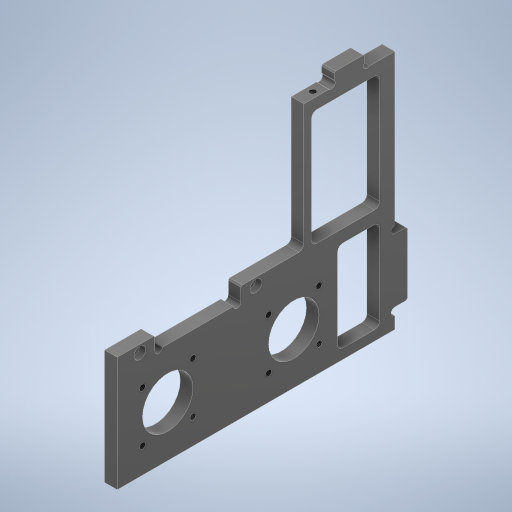
# Autodesk Inventor part: TorsoElectronicBoxSideFrame_
Saved by Autodesk Inventor 2024.2 (Build 282272000, 272)
## iProperties
Created: 2024-01-27
Part Number: TorsoElectronicBoxSideFrame_
Material: Acetal Resin, Black
Document SubType Name: Modeling
Designer: Masato Kubotera
Density: 1.425 g/cm^3
Appearance: Smooth - Black
Vendor: meviy
Mass: 39.5202 g
Surface Area: 148.13 cm^2
Volume: 27.7334 cm^3
Author: Masato Kubotera
Autodesk Inventor part; units mm, degrees
ref_plane "YZ Plane" through (0, 0, 0) normal (1, 0, 0) x (0, 1, 0)
ref_plane "XZ Plane" through (0, 0, 0) normal (0, 1, 0) x (-1, 0, 0)
ref_plane "XY Plane" through (0, 0, 0) normal (0, 0, 1) x (1, 0, 0)
derived "TorsoSideFrame_.ipt"
sketch "Sketch1" plane through (0, 0, 0) normal (0, 1, 0) x (-1, 0, 0)
  circle A0 centre (0, 0) radius 18.75
  line L0 (0, 0) -> (0, -161.5)
  circle A1 centre (0, 0) radius 29 construction
  line L1 (0, 0) -> (0, 39.5)
  line L2 (0, 39.5) -> (-47.1831, 39.5)
  line L3 (-70, -1) -> (-70, -106.5)
  line L4 (-70, -161.5) -> (-42, -161.5)
  line L5 (-42, -161.5) -> (-42, -166.5)
  line L6 (-42, -166.5) -> (-14, -166.5)
  line L7 (-14, -166.5) -> (-14, -161.5)
  line L8 (-14, -161.5) -> (0, -161.5)
  line L9 (-65, -20.95) -> (-70, -20.95)
  line L10 (-56, -161.5) -> (-56, -155.5) construction
  line L11 (-28, -166.5) -> (-28, -161.5) construction
  arc A2 (-11, -161.5) -> (-14, -161.5) centre (-12.5, -161.5) ccw
  arc A3 (-42, -161.5) -> (-45, -161.5) centre (-43.5, -161.5) ccw
  line L12 (-70, -1) -> (-65, -1) construction
  line L13 (-65, -1) -> (-65, -106.5) construction
  line L14 (-67.5, -1) -> (-67.5, -106.5) construction
  line L15 (-70, -66) -> (0, -66) construction
  line L16 (-70, -21) -> (-65, -21) construction
  arc A4 (-65, -23.95) -> (-65, -20.95) centre (-65, -22.45) ccw
  line L17 (-65, -106.5) -> (0, -106.5) construction
  line L18 (-65, -101.5) -> (0, -101.5) construction
  line L19 (-65, -104) -> (-20, -104) construction
  line L20 (-9.95, -106.55) -> (-30.05, -106.55)
  line L21 (-30.05, -106.55) -> (-30.05, -101.45)
  line L22 (-30.05, -101.45) -> (-9.95, -101.45)
  line L23 (-9.95, -101.45) -> (-9.95, -106.55)
  line L24 (-9.95, -106.55) -> (-30.05, -101.45) construction
  line L25 (-30.05, -106.55) -> (-9.95, -101.45) construction
  line L26 (-30, -101.5) -> (-30, -106.5) construction
  arc A5 (-27.05, -101.45) -> (-30.05, -101.45) centre (-28.55, -101.45) ccw
  arc A6 (-30.05, -106.55) -> (-27.05, -106.55) centre (-28.55, -106.55) ccw
  line L27 (-15, -71.5) -> (-35, -71.5) construction
  line L28 (-35, -71.5) -> (-35, -91.5) construction
  line L29 (-35, -91.5) -> (-15, -91.5) construction
  line L30 (-15, -91.5) -> (-15, -71.5) construction
  line L31 (-15, -71.5) -> (-35, -91.5) construction
  line L32 (-35, -71.5) -> (-15, -91.5) construction
  line L33 (-37.5, -69) -> (-12.5, -69)
  line L34 (-12.5, -69) -> (-12.5, -94)
  line L35 (-12.5, -94) -> (-37.5, -94)
  line L36 (-37.5, -94) -> (-37.5, -69)
  line L37 (-37.5, -69) -> (-12.5, -94) construction
  line L38 (-12.5, -69) -> (-37.5, -94) construction
  line L39 (-50, 34.5) -> (0, 34.5) construction
  line L40 (-42.05, 34.55) -> (-13.95, 34.55)
  line L41 (-13.95, 34.55) -> (-13.95, 29.45)
  line L42 (-13.95, 29.45) -> (-42.05, 29.45)
  line L43 (-42.05, 29.45) -> (-42.05, 34.55)
  line L44 (-42.05, 34.55) -> (-13.95, 29.45) construction
  line L45 (-13.95, 34.55) -> (-42.05, 29.45) construction
  line L46 (-42.05, 32) -> (-13.95, 32) construction
  line L47 (-42, 34.5) -> (-42, 29.5) construction
  line L48 (-28, 34.55) -> (-28, 29.45) construction
  line L49 (-14, 34.5) -> (-14, 29.5) construction
  arc A7 (-39.05, 34.55) -> (-42.05, 34.55) centre (-40.55, 34.55) ccw
  arc A8 (-42.05, 29.45) -> (-39.05, 29.45) centre (-40.55, 29.45) ccw
  arc A9 (-13.95, 34.55) -> (-16.95, 34.55) centre (-15.45, 34.55) ccw
  arc A10 (-16.95, 29.45) -> (-13.95, 29.45) centre (-15.45, 29.45) ccw
  line L50 (-54.4689, -111.271) -> (-4.7987, -153.6833)
  line L51 (-65.9501, -109.75) -> (-65.9501, -154.5)
  line L52 (-63.9501, -156.5) -> (-11.5422, -156.5)
  line L53 (-10.2434, -152.979) -> (-62.6514, -108.229)
  arc A11 (-62.6514, -108.229) -> (-65.9501, -109.75) centre (-63.9501, -109.75) ccw
  arc A12 (-65.9501, -154.5) -> (-63.9501, -156.5) centre (-63.9501, -154.5) ccw
  arc A13 (-11.5422, -156.5) -> (-10.2434, -152.979) centre (-11.5422, -154.5) ccw
  line L54 (-61.4895, -100.25) -> (-33.6254, -100.25)
  circle A14 centre (-46.25, -59) radius 3 construction
  line L55 (-1.5, -56) -> (-61.4895, -56)
  line L56 (0, 0) -> (-29, 0) construction
  line L57 (-40.95, 23.9454) -> (-40.95, -23.9454)
  line L58 (-53.1702, -107.75) -> (-33.6254, -107.75)
  arc A15 (-31.9336, -108.6833) -> (-25.8669, -109.5167) centre (-28.55, -106.55) ccw
  line L59 (-1.5, -152.1623) -> (-1.5, -109.75)
  arc A16 (-53.1702, -107.75) -> (-54.4689, -111.271) centre (-53.1702, -109.75) ccw
  arc A17 (-1.5, -109.75) -> (-3.5, -107.75) centre (-3.5, -109.75) ccw
  arc A18 (-31.9336, -108.6833) -> (-33.6254, -107.75) centre (-33.6254, -109.75) ccw
  circle A19 centre (-36, -104) radius 1.75 construction
  arc A20 (-24.5254, -109) -> (-25.8669, -109.5167) centre (-24.5254, -111) ccw
  line L60 (-47.1831, 39.5) -> (-70, -1)
  line L61 (-46.582, -26.0941) -> (-61.4895, -26.0941)
  line L62 (-20, -101.45) -> (-20, -106.55) construction
  arc A21 (-33.6254, -100.25) -> (-31.9336, -99.3167) centre (-33.6254, -98.25) ccw
  arc A22 (-25.8669, -98.4833) -> (-31.9336, -99.3167) centre (-28.55, -101.45) ccw
  arc A23 (-25.8669, -98.4833) -> (-24.5254, -99) centre (-24.5254, -97) ccw
  line L63 (-10, -101.5) -> (-10, -106.5) construction
  arc A24 (-12.95, -106.55) -> (-9.95, -106.55) centre (-11.45, -106.55) ccw
  arc A25 (-6.3746, -107.75) -> (-8.0664, -108.6833) centre (-6.3746, -109.75) ccw
  arc A26 (-14.1331, -109.5167) -> (-15.4746, -109) centre (-15.4746, -111) ccw
  arc A27 (-14.1331, -109.5167) -> (-8.0664, -108.6833) centre (-11.45, -106.55) ccw
  arc A28 (-9.95, -101.45) -> (-12.95, -101.45) centre (-11.45, -101.45) ccw
  arc A29 (-15.4746, -99) -> (-14.1331, -98.4833) centre (-15.4746, -97) ccw
  arc A30 (-8.0664, -99.3167) -> (-14.1331, -98.4833) centre (-11.45, -101.45) ccw
  arc A31 (-8.0664, -99.3167) -> (-6.3746, -100.25) centre (-6.3746, -98.25) ccw
  line L64 (-24.5254, -99) -> (-15.4746, -99)
  line L65 (-24.5254, -109) -> (-15.4746, -109)
  line L66 (-6.3746, -107.75) -> (-3.5, -107.75)
  line L67 (-6.3746, -100.25) -> (-3.5, -100.25)
  arc A32 (-3.5, -100.25) -> (-1.5, -98.25) centre (-3.5, -98.25) ccw
  line L68 (-46.25, -59) -> (-41.25, -59) construction
  line L69 (-65, -23.95) -> (-65, -78.05)
  line L70 (-65, -51) -> (-70, -51) construction
  line L71 (-70, -81) -> (-65, -81) construction
  arc A33 (-65, -81.05) -> (-65, -78.05) centre (-65, -79.55) ccw
  line L72 (-65, -81.05) -> (-70, -81.05)
  line L73 (-65, -106.5) -> (-70, -106.5) construction
  line L74 (-1.5, -22.4499) -> (-1.5, -56)
  line L75 (-61.4895, -62) -> (-1.5, -62)
  line L76 (-1.5, -62) -> (-1.5, -98.25)
  line L77 (-61.4895, -56) -> (-61.4895, -26.0941)
  circle A34 centre (-25, -81.5) radius 10
  line L78 (-61.4895, -62) -> (-61.4895, -100.25)
  arc A35 (-4.7987, -153.6833) -> (-1.5, -152.1623) centre (-3.5, -152.1623) ccw
  circle A36 centre (-25, -81.5) radius 11
  arc A37 (-14.0872, 17.5443) -> (-22.2374, 3.4277) centre (0, 0) ccw
  arc A38 (-22.2374, -3.4277) -> (-14.0872, -17.5443) centre (0, 0) ccw
  arc A39 (-8.1502, -20.972) -> (-1.5, -22.4499) centre (0, 0) ccw
  arc A40 (-14.0872, -17.5443) -> (-8.1502, -20.972) centre (-12.375, -21.4341) ccw
  arc A41 (-22.2374, 3.4277) -> (-22.2374, -3.4277) centre (-24.75, 0) ccw
  arc A42 (-10.9839, 25.45) -> (-14.0872, 17.5443) centre (-12.375, 21.4341) ccw
  line L79 (-70, -106.5) -> (-70, -161.5)
  point P0 (-16.05, -9.6933)
  point P1 (12.375, -21.4341)
  point P2 (24.75, 0)
  point P3 (12.375, 21.4341)
  point P4 (-70, -66)
  point P5 (0, -66)
  point P6 (-47.5, -132.5)
  point P7 (-28, 32)
  point P8 (0, -130.75)
  point P9 (-45.6341, -118.8149)
  point P10 (0, -157.7808)
  point P11 (-48, 32)
  point P12 (-53.9811, -94)
  point P13 (-1.5, -156.5)
  point P14 (-7, -161.5)
  point P15 (-66.3533, -107.75)
  point P16 (-32.3658, -107.75)
  point P17 (-32.5089, -107.1221)
  point P18 (-7.6342, -107.75)
  point P19 (-42, 32)
sketch "Sketch2" plane through (0, 0, 0) normal (0, 1, 0) x (-1, 0, 0)
  arc A0 (65, -93.75) -> (65, -96.75) centre (65, -95.25) ccw
  line L0 (65, -99.75) -> (59, -99.75) construction
  line L1 (70, -93.75) -> (65, -93.75)
  line L2 (65, -93.75) -> (65, -101.5)
  line L3 (65, -62.75) -> (59, -62.75) construction
  line L4 (65, -1) -> (65, -68.75)
  line L5 (70, -81.25) -> (65, -81.25) construction
  line L6 (65, -68.75) -> (70, -68.75)
  line L7 (70, -68.75) -> (70, -93.75)
  arc A1 (65, -65.75) -> (65, -68.75) centre (65, -67.25) ccw
  line L8 (65, -101.5) -> (-45, -101.5)
  line L9 (-45, -101.5) -> (-45, -56)
  line L10 (29, -56) -> (29, -1)
  line L11 (29, -1) -> (65, -1)
  line L12 (29, -6) -> (41, -6)
  line L13 (41, -6) -> (41, -1)
  line L14 (53, -1) -> (53, -6)
  line L15 (53, -6) -> (65, -6)
  line L16 (47, -1) -> (47, -6) construction
  arc A2 (38.8787, -6) -> (41, -3.8787) centre (39.9393, -4.9393) ccw
  line L17 (35, -6) -> (35, -12) construction
  arc A3 (53, -3.8787) -> (55.1213, -6) centre (54.0607, -4.9393) ccw
  line L18 (-30, -56.5) -> (4, -56.5) construction
  line L19 (4, -56.5) -> (4, -61.5) construction
  line L20 (4, -61.5) -> (-30, -61.5) construction
  line L21 (-30, -61.5) -> (-30, -56.5) construction
  line L22 (-30, -56.5) -> (4, -61.5) construction
  line L23 (4, -56.5) -> (-30, -61.5) construction
  line L24 (-30, -59) -> (4, -59) construction
  line L25 (-13, -56.5) -> (-13, -61.5) construction
  line L26 (4.05, -61.55) -> (-30.05, -61.55)
  line L27 (-30.05, -61.55) -> (-30.05, -56)
  line L28 (4.05, -56) -> (4.05, -61.55)
  arc A4 (-30.05, -61.55) -> (-27.05, -61.55) centre (-28.55, -61.55) ccw
  arc A5 (1.05, -61.55) -> (4.05, -61.55) centre (2.55, -61.55) ccw
  line L29 (-65, -1) -> (-65, -106.5) construction
  line L30 (0, 0) -> (0, -161.5) construction
  line L31 (65, -1) -> (65, -106.5) construction
  line L32 (-70, -66) -> (0, -66) construction
  line L33 (-65, -101.5) -> (0, -101.5) construction
  line L34 (-37.5, -69) -> (-12.5, -69) construction
  line L35 (-12.5, -69) -> (-12.5, -94) construction
  line L36 (-37.5, -94) -> (-37.5, -69) construction
  line L37 (-12.5, -94) -> (-37.5, -94) construction
  arc A6 (-37.5, -71.5) -> (-35, -69) centre (-35, -71.5) ccw
  arc A7 (-35, -94) -> (-37.5, -91.5) centre (-35, -91.5) ccw
  arc A8 (-12.5, -91.5) -> (-15, -94) centre (-15, -91.5) ccw
  arc A9 (-15, -69) -> (-12.5, -71.5) centre (-15, -71.5) ccw
  line L38 (-37.5, -71.5) -> (-37.5, -91.5)
  line L39 (-35, -94) -> (-15, -94)
  line L40 (-12.5, -91.5) -> (-12.5, -71.5)
  line L41 (-15, -69) -> (-35, -69)
  line L42 (37.5, -69) -> (12.5, -69) construction
  line L43 (12.5, -69) -> (12.5, -94) construction
  line L44 (37.5, -94) -> (37.5, -69) construction
  line L45 (12.5, -94) -> (37.5, -94) construction
  arc A10 (35, -69) -> (37.5, -71.5) centre (35, -71.5) ccw
  arc A11 (37.5, -91.5) -> (35, -94) centre (35, -91.5) ccw
  arc A12 (15, -94) -> (12.5, -91.5) centre (15, -91.5) ccw
  arc A13 (12.5, -71.5) -> (15, -69) centre (15, -71.5) ccw
  line L46 (37.5, -71.5) -> (37.5, -91.5)
  line L47 (35, -94) -> (15, -94)
  line L48 (12.5, -91.5) -> (12.5, -71.5)
  line L49 (15, -69) -> (35, -69)
  line L50 (-70, -1) -> (-65, -1) construction
  line L51 (32, -10.5) -> (32, -56.5)
  line L52 (32, -56.5) -> (59, -56.5)
  line L53 (59, -56.5) -> (59, -10.5)
  line L54 (59, -10.5) -> (32, -10.5)
  line L55 (-45, -56) -> (-30.05, -56)
  line L56 (29, -56) -> (4.05, -56)
  line L57 (42.3365, -61.5) -> (59, -61.5)
  line L58 (59, -61.5) -> (59, -97.5894)
  line L59 (59, -97.5894) -> (42.3365, -97.5894)
  line L60 (42.3365, -97.5894) -> (42.3365, -61.5)
  circle A14 centre (-25, -81.5) radius 10 projected
  circle A15 centre (25, -81.5) radius 10
  point P0 (-13, -59)
  point P1 (-36, -59)
  point P2 (10, -59)
  point P3 (-35, -71.5)
  point P4 (-35, -91.5)
  point P5 (-15, -91.5)
  point P6 (-15, -71.5)
  point P7 (4.05, -61.55)
  point P8 (1.05, -61.55)
  point P9 (-30.05, -61.55)
  point P10 (-30.05, -61.55)
  point P11 (65, -96.75)
  point P12 (55.1213, -6)
  point P13 (53, -3.8787)
  dimension "d1" = 25
  dimension "d2" = 6
  dimension "d3" = 1.5
  dimension "d5" = 6
  dimension "d7" = 5
  dimension "d8" = 6
  dimension "d9" = 6
  dimension "d11" = 5
  dimension "d13" = 0.05
  dimension "d15" = 6
  dimension "d19" = 35
  dimension "d20" = 20
  dimension "d21" = 40
  dimension "d22" = 5
  dimension "d23" = 34
  dimension "d24" = 36
  dimension "d64" = 3
  dimension "d65" = 12
  dimension "d66" = 0.05
  dimension "d67" = 5.5
  dimension "d68" = 4.5
  dimension "d69" = 100.5
  dimension "d70" = 160.5
  constraints: 104 end point, 34 symmetric about line, 32 point on line, 29 point on circle, 15 centre point, 13 horizontal, 9 midpoint, 8 coincident, 8 collinear, 8 vertical, 6 tangent, 5 perpendicular, 4 parallel, 2 equal radius, 11 other
  measures "d1" distance of L7.start L7.end
  measures "d2" distance of L3.start L3.end
  measures "d3" radius of A1
  measures "d5" distance between parallel lines of L3 L6
  measures "d7" distance between parallel lines of L12 L11
  measures "d8" distance of L17.start L17.end
  measures "d9" distance between parallel lines of L13 L17
  measures "d11" distance of L18.end L20.start
  measures "d13" distance between parallel lines of L27 L21
  measures "d15" distance from line of point (-36, -59) L21
  measures "d19" distance between parallel lines of L21 L29
  measures "d20" distance between parallel lines of L29 L9
  measures "d21" distance between parallel lines of L8 L20
  measures "d22" distance of L7.end L2.start
  measures "d23" distance between parallel lines of L21 L19
  measures "d24" distance of L11.start L4.start
  measures "d64" distance between parallel lines of L10 L51
  measures "d65" distance between parallel lines of L10 L13
  measures "d66" distance between parallel lines of L26 L20
  measures "d67" distance between parallel lines of L20 L56
  measures "d68" distance between parallel lines of L54 L12
  measures "d69" distance between parallel lines of L8 L11
  measures "d70" diameter of L11 L5
extrude "Extrusion1" add sketch "Sketch2" against normal blind 5 contours A0 L2 L8 L9 L55 L27 A4 L26 A5 L28 L56 L10 L12 A2 L13 L11 L14 A3 L15 L4 A1 L6 L7 L1 | A6 L41 A9 L40 A8 L39 A7 L38 | A10 L46 A11 L47 A12 L48 A13 L49
hole "Phi3.5" at (35, 0, -71.5) at (35, 0, -91.5) at (15, 0, -91.5) at (15, 0, -71.5) at (-15, 0, -71.5) at (-15, 0, -91.5) at (-35, 0, -91.5) at (-35, 0, -71.5) direction (0, -1, 0) diameter 2.459 end through all thread size "M3x0.5" class "6H" standard "ANSI Metric M Profile"
hole "Phi2.5" at (36, 0, -59) at (-10, 0, -59) direction (0, -1, 0) diameter 2.5 end through all counterbore diameter 4.8 counterbore depth 2.5
chamfer "Chamfer1" distance 0.5 angle 45 6 edges at (-53, -2.5, -1) (-41, -2.5, -1) (-70, -2.5, -68.75) (-70, -2.5, -93.75) (30.05, -2.5, -56) (-4.05, -2.5, -56)
sketch "Sketch3" plane through (-65, 0, -65.75) normal (-1, 0, 0) x (0, 0, -1)
  line L0 (3, 5) -> (0, 5) projected
  line L1 (-3, 5) -> (-3, 0)
  line L2 (28, 5) -> (35.75, 5) projected
  line L3 (34, 5) -> (34, 0)
  point P0 (-65.75, 0)
  point P1 (-59.75, 5)
  point P2 (31, 5)
  point P3 (-3, 0)
  point P4 (-3, 0)
  point P5 (-3, 0)
  point P6 (34, 0)
  point P7 (34, 0)
  point P8 (34, 0)
  point P9 (-3, 2.5)
  point P10 (34, 2.5)
  point P11 (-49.5, 5)
  constraints: 4 end point, 2 coincident, 2 midpoint, 2 point on line, 2 vertical
hole "Hole3" at (-65, -2.5, -62.75) at (-65, -2.5, -99.75) direction (1, 0, 0) diameter 2.459 depth 6 thread size "M3x0.5" class "6H" standard "ANSI Metric M Profile"
sketch "Sketch4" plane through (-38.8787, 0, -6) normal (0, 0, 1) x (-1, 0, 0)
  line L0 (-9.8787, 5) -> (0, 5) projected
  line L1 (-3.8787, 5) -> (-3.8787, 0)
  point P0 (-38.8787, 0)
  point P1 (-3.8787, 0)
  point P2 (-3.8787, 0)
  point P3 (-3.8787, 2.5)
  constraints: 2 end point, 1 coincident, 1 midpoint, 1 point on line, 1 vertical
hole "Hole4" at (-35, -2.5, -6) direction (0, 0, -1) diameter 2.459 depth 6 thread size "M3x0.5" class "6H" standard "ANSI Metric M Profile"
fillet "Fillet1" radius 2 9 edges at (-29, -2.5, -56) (-32, -2.5, -10.5) (-59, -2.5, -10.5) (-32, -2.5, -56.5) (-59, -2.5, -56.5) (-59, -2.5, -61.5) (-42.3365, -2.5, -61.5) (-42.3365, -2.5, -97.5894) (-59, -2.5, -97.5894)
equation "\"d49\" = d2"
equation "\"d56\" = d8"
body "Solid1"
